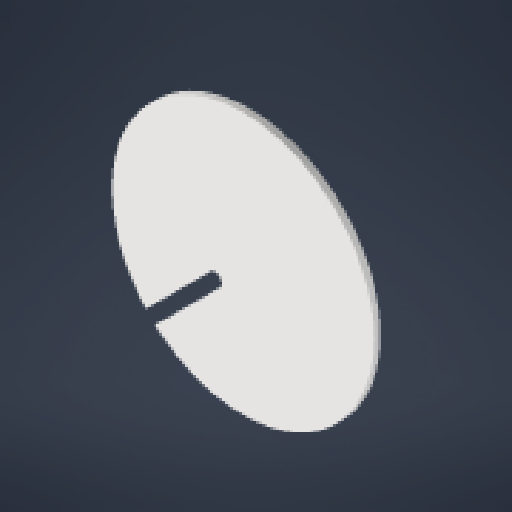
# Autodesk Inventor part: drehkranz 2
Saved by Autodesk Inventor 2023 (Build 270158000, 158)
## iProperties
Created: 2026-03-19
Part Number: drehkranz 2
Material: Generisch
Document SubType Name: Modeling
Designer: lerat
Mass: 162.042 g
Surface Area: 678.095 cm^2
Volume: 162.042 cm^3
Density: 1 g/cm^3
Appearance: Vorgabe
Author: lerat
Autodesk Inventor part; units mm, degrees
ref_plane "YZ Plane" through (0, 0, 0) normal (1, 0, 0) x (0, 1, 0)
ref_plane "XZ Plane" through (0, 0, 0) normal (0, 1, 0) x (-1, 0, 0)
ref_plane "XY Plane" through (0, 0, 0) normal (0, 0, 1) x (1, 0, 0)
sketch "Skizze1" plane through (0, 0, 0) normal (0, 0, 1) x (1, 0, 0)
  circle A0 centre (0, 0) radius 100
  line L0 (0, 0) -> (0, 92.5)
  circle A1 centre (0, 92.5) radius 4.6
  circle A2 centre (-92.5, 0) radius 4.6
  circle A3 centre (0, -92.5) radius 4.6
  circle A4 centre (92.5, 0) radius 4.6
  dimension "d0" = 200
  dimension "d1" = 92.5
  dimension "d2" = 9.2
  dimension "d5" = 360
  constraints: 5 centre point, 2 coincident, 2 end point, 1 vertical, 9 other
  measures "d0" diameter of A0
  measures "d1" distance of L0.start L0.end
  measures "d2" diameter of A1
extrude "Extrusion1" add sketch "Skizze1" along normal blind 4
sketch "Skizze2" plane through (0, 0, 0) normal (0, 0, -1) x (-1, 0, 0)
  circle A0 centre (0, 0) radius 9
  dimension "d9" = 18
  constraints: 1 centre point, 1 coincident
  measures "d9" diameter of A0
extrude "Extrusion2" add sketch "Skizze2" along normal blind 14.8
sketch "Skizze3" plane through (0, 0, -14.8) normal (0, 0, -1) x (-1, 0, 0)
  circle A0 centre (0, 0) radius 2.5
  point P0 (0, 0)
  constraints: 1 centre point, 2 other
extrude "Extrusion3" cut sketch "Skizze3" against normal through all
sketch "Skizze4" plane through (0, 0, -14.8) normal (0, 0, -1) x (-1, 0, 0)
  line L0 (4.2499, 4.1103) -> (-4.6053, 4.1103)
  line L1 (-4.6053, 4.1103) -> (-4.6053, 1.6)
  line L2 (-4.6053, 1.6) -> (4.2499, 1.6)
  line L3 (4.2499, 1.6) -> (4.2499, 4.1103)
  line L4 (3.4775, -2.7862) -> (-3.9432, -2.7862)
  line L5 (-3.9432, -2.7862) -> (-3.9432, -1.6)
  line L6 (-3.9432, -1.6) -> (3.4775, -1.6)
  line L7 (3.4775, -1.6) -> (3.4775, -2.7862)
  point P0 (0, 0)
  dimension "d14" = 3.2
  dimension "d15" = 1.6
  constraints: 16 end point, 4 parallel, 2 horizontal, 2 perpendicular
  measures "d14" distance between parallel lines of L6 L2
  measures "d15" distance from line of L2 point (0, 0)
extrude "Extrusion4" add sketch "Skizze4" against normal up to surface (18.8 mm away)
sketch "Skizze5" plane through (0, 0, 4) normal (0, 0, 1) x (1, 0, 0)
  circle A0 centre (0, 0) radius 100 projected
extrude "Extrusion5" add sketch "Skizze5" along normal blind 1
sketch "Skizze6" plane through (0, 0, 5) normal (0, 0, 1) x (1, 0, 0)
  line L0 (-73.8057, -80.8768) -> (-14.1421, -21.2132)
  line L1 (-14.1421, -21.2132) -> (-21.2132, -14.1421)
  line L2 (-21.2132, -14.1421) -> (-80.8768, -73.8057)
  line L3 (-80.8768, -73.8057) -> (-73.8057, -80.8768)
  line L4 (-77.3412, -77.3412) -> (0, 0) construction
  line L5 (0, 0) -> (0, -95.3609) construction
  point P0 (-17.6777, -17.6777)
  dimension "d21" = 45
  dimension "d22" = 10
  dimension "d23" = 25
  constraints: 12 end point, 2 midpoint, 2 parallel, 1 perpendicular, 1 point on line, 1 vertical
  measures "d21" angle of L5 L4
  measures "d22" distance between parallel lines of L2 L0
  measures "d23" distance from line of L4.end L1
extrude "Extrusion6" cut sketch "Skizze6" against normal blind 5
fillet "Rundung1" radius 5 2 edges at (-14.1421, -21.2132, 2.5) (-21.2132, -14.1421, 2.5)
fillet "Rundung2" radius 5 3 edges at (-16.213, -21.2132, 0) (-49.4531, -42.382, 0) (-42.382, -49.4531, 0)
equation "\"d15\" = 0.5 * d14"
